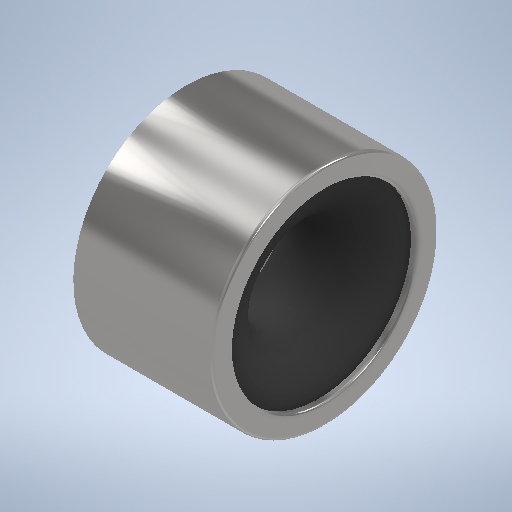
# Autodesk Inventor part: AirBagV1
Saved by Autodesk Inventor 2025.2 (Build 292293000, 293)
## iProperties
Created: 2025-08-30
Part Number: AirBagV1
Material: Steel, Alloy
Document SubType Name: Modeling
Designer: aaron
Density: 7.73 g/cm^3
Appearance: Semi-Polished
Author: aaron
Autodesk Inventor part; units mm, degrees
ref_plane "YZ Plane" through (0, 0, 0) normal (1, 0, 0) x (0, 1, 0)
ref_plane "XZ Plane" through (0, 0, 0) normal (0, 1, 0) x (-1, 0, 0)
sketch "Sketch1" plane through (0, 0, 0) normal (1, 0, 0) x (0, 1, 0)
  circle A0 centre (0, 0) radius 88.9
  circle A1 centre (0, 0) radius 92.075
  dimension "d0" = 177.8
  dimension "d1" = 184.15
  constraints: 2 centre point, 2 coincident
  measures "d0" diameter of A0
  measures "d1" diameter of A1
extrude "Extrusion1" add sketch "Sketch1" along normal blind 101.6
ref_plane "Work Plane1" through (50.8, 0, 0) normal (1, 0, 0) x (0, 0, -1)
sketch "Sketch5" plane through (0, 0, 0) normal (0, 1, 0) x (-1, 0, 0)
  line L0 (20.32, 0) -> (-121.92, 0) projected
  line L1 (0, -88.9) -> (0, 88.9) projected
  line L2 (0, 88.9) -> (-101.6, 88.9)
  line L3 (-101.6, 92.075) -> (-101.6, -92.075) projected
  line L4 (-101.6, -88.9) -> (-101.6, 88.9) projected
  arc A0 (-101.6, 88.9) -> (0, 88.9) centre (-50.8, 88.9) ccw
  point P0 (0, 0)
  dimension "d23" = 50.8
  constraints: 2 end point, 2 point on circle, 1 centre point, 1 horizontal, 1 point on line
  measures "d23" radius of A0
revolve "Revolution1" add sketch "Sketch5" angle 360 about axis through (-10, 0, 0) along (1, 0, 0) contours A0 L2
sketch "Sketch6" plane through (0, 0, 0) normal (1, 0, 0) x (0, 1, 0)
  circle A0 centre (0, 0) radius 104.775
  circle A1 centre (0, 0) radius 107.95
  dimension "d17" = 215.9
  dimension "d18" = 209.55
  constraints: 2 centre point, 2 coincident
  measures "d17" diameter of A1
  measures "d18" diameter of A0
extrude "Extrusion3" add sketch "Sketch6" along normal blind 101.6 and the other way blind 25.4
sketch "Sketch7" plane through (101.6, 0, 0) normal (1, 0, 0) x (0, 0, -1)
  circle A0 centre (0, 0) radius 107.95
  circle A1 centre (0, 0) radius 87.7627
  constraints: 2 centre point, 2 coincident
extrude "Extrusion4" add sketch "Sketch7" along normal blind 6.35
fillet "Fillet1" radius 3.175 2 edges at (107.95, 0, 87.7627) (107.95, 0, 107.95)
body "Solid1"
